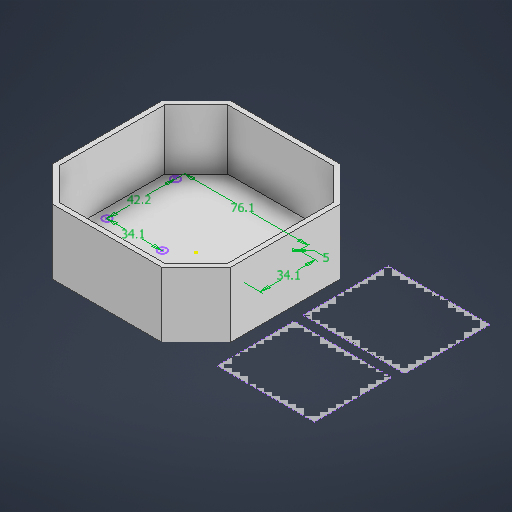
# Autodesk Inventor part: GPS-Compass_box
Saved by Autodesk Inventor 2026.1 (Build 301233020, 233B)
## iProperties
Created: 2025-11-10
Part Number: GPS-Compass_box
Material: Generic
Document SubType Name: Modeling
Designer: MenMe
Density: 1 g/cm^3
Appearance: Default
Author: MenMe
Autodesk Inventor part; units mm, degrees
ref_plane "YZ Plane" through (0, 0, 0) normal (1, 0, 0) x (0, 1, 0)
ref_plane "XZ Plane" through (0, 0, 0) normal (0, 1, 0) x (-1, 0, 0)
ref_plane "XY Plane" through (0, 0, 0) normal (0, 0, 1) x (1, 0, 0)
sketch "Sketch1" plane through (0, 0, 0) normal (0, 1, 0) x (-1, 0, 0)
  line L0 (-55, 0) -> (55, 0) construction
  line L1 (0, 55) -> (0, -55) construction
  line L2 (55, 33.7868) -> (55, -33.7868)
  line L3 (55, 33.7868) -> (33.7868, 55)
  line L4 (33.7868, 55) -> (-33.7868, 55)
  line L5 (-33.7868, 55) -> (-55, 33.7868)
  line L6 (-55, 33.7868) -> (-55, -33.7868)
  line L7 (-55, -33.7868) -> (-33.7868, -55)
  line L8 (-33.7868, -55) -> (33.7868, -55)
  line L9 (33.7868, -55) -> (55, -33.7868)
  point P0 (0, 0)
  point P1 (0, 0)
  point P2 (55, 0)
  dimension "d0" = 110
  dimension "d1" = 110
  dimension "d2" = 135
  dimension "d3" = 135
  dimension "d4" = 135
  dimension "d8" = 30
  constraints: 20 end point, 7 midpoint, 2 horizontal, 2 perpendicular, 2 vertical, 1 coincident, 1 parallel
  measures "d0" distance of L0.start L0.end
  measures "d1" distance of L1.start L1.end
  measures "d2" angle of L2 L3
  measures "d3" angle of L2 L9
  measures "d4" angle of L5 L6
  measures "d8" distance of L6.end L7.end
extrude "Extrusion1" add sketch "Sketch1" along normal blind 40
sketch "Sketch2" plane through (0, 40, 0) normal (0, 1, 0) x (1, 0, 0)
  line L0 (33.7868, -55) -> (55, -33.7868) projected
  line L1 (55, -33.7868) -> (55, 33.7868) projected
  line L2 (55, 33.7868) -> (33.7868, 55) projected
  line L3 (33.7868, 55) -> (-33.7868, 55) projected
  line L4 (-33.7868, 55) -> (-55, 33.7868) projected
  line L5 (-55, 33.7868) -> (-55, -33.7868) projected
  line L6 (-55, -33.7868) -> (-33.7868, -55) projected
  line L7 (-33.7868, -55) -> (33.7868, -55) projected
  line L8 (-32.5442, 52) -> (32.5442, 52)
  line L9 (32.5442, 52) -> (52, 32.5442)
  line L10 (52, 32.5442) -> (52, -32.5442)
  line L11 (52, -32.5442) -> (32.5442, -52)
  line L12 (32.5442, -52) -> (-32.5442, -52)
  line L13 (-32.5442, -52) -> (-52, -32.5442)
  line L14 (-52, -32.5442) -> (-52, 32.5442)
  line L15 (-52, 32.5442) -> (-32.5442, 52)
  point P0 (0, 0)
  dimension "d11" = 3
  constraints: 16 end point, 7 other
  measures "d11" distance between parallel lines of L3 L8
extrude "Extrusion2" cut sketch "Sketch2" against normal blind 37 contours L8 L9 L10 L11 L12 L13 L14 L15
sketch "Sketch3" plane through (0, 3, 0) normal (0, 1, 0) x (1, 0, 0)
  line L0 (65.7305, 52.5845) -> (128.5575, 52.5845) construction
  line L1 (128.5575, 52.5845) -> (128.5575, -0.1453) construction
  line L2 (128.5575, -0.1453) -> (65.7305, -0.1453) construction
  line L3 (65.7305, -0.1453) -> (65.7305, 52.5845) construction
  circle A0 centre (-46.0713, 33.2689) radius 2.5
  circle A1 centre (-46.0713, -8.9311) radius 2.5
  circle A2 centre (-11.9713, -8.9311) radius 2.5
  circle A3 centre (30.0287, 33.2689) radius 2.5
  circle A4 centre (30.0287, -0.8311) radius 2.5
  line L4 (66.173, -5.8852) -> (126.4692, -5.8852) construction
  line L5 (126.4692, -5.8852) -> (126.4692, -53.6631) construction
  line L6 (126.4692, -53.6631) -> (66.173, -53.6631) construction
  line L7 (66.173, -53.6631) -> (66.173, -5.8852) construction
  point P0 (0, 0)
  dimension "d40" = 5
  dimension "d43" = 34.1
  dimension "d58" = 76.1
  dimension "d59" = 42.2
  dimension "d60" = 34.1
  constraints: 5 centre point, 4 equal radius, 2 horizontal alignment, 2 vertical alignment, 4 other
  measures "d40" diameter of A3
  measures "d43" distance of A3.centre A4.centre
  measures "d58" distance of A0.centre A3.centre
  measures "d59" distance of A1.centre A0.centre
  measures "d60" distance of A2.centre A1.centre
body "Solid1"
